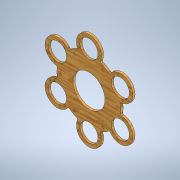
# Autodesk Inventor part: AmmoHolder
Saved by Autodesk Inventor 2020.2 (Build 242310000, 310)
## iProperties
Created: 2019-11-06
Part Number: AmmoHolder
Material: Plywood, Finish
Document SubType Name: Modeling
Designer: Paul Lefeuvre
Density: 0.552 g/cm^3
Appearance: Plywood - New
Mass: 279.601 g
Surface Area: 1409.01 cm^2
Volume: 506.524 cm^3
Author: Paul Lefeuvre
Autodesk Inventor part; units mm, degrees
ref_plane "YZ Plane" through (0, 0, 0) normal (1, 0, 0) x (0, 1, 0)
ref_plane "XZ Plane" through (0, 0, 0) normal (0, 1, 0) x (-1, 0, 0)
ref_plane "XY Plane" through (0, 0, 0) normal (0, 0, 1) x (1, 0, 0)
sketch "Sketch3" plane through (0, 0, 0) normal (0, 0, 1) x (1, 0, 0)
  circle A0 centre (0, 0) radius 191.2 construction
  circle A1 centre (0, 153.1) radius 37.5 construction
  circle A2 centre (0, 153.1) radius 38.1
  line L0 (0, 0) -> (0, 212.7207) construction
  arc A3 (48.5367, 131.5641) -> (-48.5367, 131.5641) centre (0, 153.1) ccw
  arc A4 (-51.2104, 124.91) -> (-48.5367, 131.5641) centre (-53.1071, 129.5363) ccw
  arc A5 (48.5367, 131.5641) -> (51.2104, 124.91) centre (53.1071, 129.5363) ccw
  circle A6 centre (-132.5885, 76.55) radius 38.1
  arc A7 (-89.6695, 107.8161) -> (-138.2062, 23.748) centre (-132.5885, 76.55) ccw
  arc A8 (-133.7804, 18.1055) -> (-138.2062, 23.748) centre (-138.7352, 18.7761) ccw
  arc A9 (-89.6695, 107.8161) -> (-82.57, 106.8045) centre (-85.6282, 110.7602) ccw
  circle A10 centre (-132.5885, -76.55) radius 38.1
  arc A11 (-138.2062, -23.748) -> (-89.6695, -107.8161) centre (-132.5885, -76.55) ccw
  arc A12 (-82.57, -106.8045) -> (-89.6695, -107.8161) centre (-85.6282, -110.7602) ccw
  arc A13 (-138.2062, -23.748) -> (-133.7804, -18.1055) centre (-138.7352, -18.7761) ccw
  circle A14 centre (0, -153.1) radius 38.1
  arc A15 (-48.5367, -131.5641) -> (48.5367, -131.5641) centre (0, -153.1) ccw
  arc A16 (51.2104, -124.91) -> (48.5367, -131.5641) centre (53.1071, -129.5363) ccw
  arc A17 (-48.5367, -131.5641) -> (-51.2104, -124.91) centre (-53.1071, -129.5363) ccw
  circle A18 centre (132.5885, -76.55) radius 38.1
  arc A19 (89.6695, -107.8161) -> (138.2062, -23.748) centre (132.5885, -76.55) ccw
  arc A20 (133.7804, -18.1055) -> (138.2062, -23.748) centre (138.7352, -18.7761) ccw
  arc A21 (89.6695, -107.8161) -> (82.57, -106.8045) centre (85.6282, -110.7602) ccw
  circle A22 centre (132.5885, 76.55) radius 38.1
  arc A23 (138.2062, 23.748) -> (89.6695, 107.8161) centre (132.5885, 76.55) ccw
  arc A24 (82.57, 106.8045) -> (89.6695, 107.8161) centre (85.6282, 110.7602) ccw
  arc A25 (138.2062, 23.748) -> (133.7804, 18.1055) centre (138.7352, 18.7761) ccw
  arc A26 (-51.2104, 124.91) -> (-82.57, 106.8045) centre (0, 0) ccw
  arc A27 (82.57, 106.8045) -> (51.2104, 124.91) centre (0, 0) ccw
  arc A28 (133.7804, -18.1055) -> (133.7804, 18.1055) centre (0, 0) ccw
  arc A29 (51.2104, -124.91) -> (82.57, -106.8045) centre (0, 0) ccw
  arc A30 (-82.57, -106.8045) -> (-51.2104, -124.91) centre (0, 0) ccw
  arc A31 (-133.7804, 18.1055) -> (-133.7804, -18.1055) centre (0, 0) ccw
  circle A32 centre (41.5415, 141.1) radius 3.3
  line L1 (0, 153.1) -> (41.5415, 141.1) construction
  circle A33 centre (41.5415, 165.1) radius 3.3
  line L2 (0, 153.1) -> (41.5415, 165.1) construction
  line L3 (41.5415, 141.1) -> (41.5415, 165.1) construction
  circle A34 centre (-41.5415, 141.1) radius 3.3
  circle A35 centre (-41.5415, 165.1) radius 3.3
  circle A36 centre (-163.7516, 46.574) radius 3.3
  circle A37 centre (-142.9669, 34.574) radius 3.3
  circle A38 centre (-122.21, 118.526) radius 3.3
  circle A39 centre (-101.4254, 106.526) radius 3.3
  circle A40 centre (-122.21, -118.526) radius 3.3
  circle A41 centre (-101.4254, -106.526) radius 3.3
  circle A42 centre (-163.7516, -46.574) radius 3.3
  circle A43 centre (-142.9669, -34.574) radius 3.3
  circle A44 centre (41.5415, -165.1) radius 3.3
  circle A45 centre (41.5415, -141.1) radius 3.3
  circle A46 centre (-41.5415, -165.1) radius 3.3
  circle A47 centre (-41.5415, -141.1) radius 3.3
  circle A48 centre (163.7516, -46.574) radius 3.3
  circle A49 centre (142.9669, -34.574) radius 3.3
  circle A50 centre (122.21, -118.526) radius 3.3
  circle A51 centre (101.4254, -106.526) radius 3.3
  circle A52 centre (122.21, 118.526) radius 3.3
  circle A53 centre (101.4254, 106.526) radius 3.3
  circle A54 centre (163.7516, 46.574) radius 3.3
  circle A55 centre (142.9669, 34.574) radius 3.3
  circle A56 centre (0, 0) radius 100 construction
  circle A57 centre (0, 0) radius 72.5 construction
  circle A58 centre (0, 0) radius 67.5
  line L4 (0, 0) -> (-241.025, 0) construction
  circle A59 centre (-120, 0) radius 3.9
  line L5 (0, 0) -> (-120.5125, -208.7337) construction
  circle A60 centre (-60, -103.923) radius 3.9
  line L6 (0, 0) -> (120.5125, -208.7337) construction
  circle A61 centre (60, -103.923) radius 3.9
  line L7 (0, 0) -> (241.025, 0) construction
  circle A62 centre (120, 0) radius 3.9
  line L8 (0, 0) -> (120.5125, 208.7337) construction
  circle A63 centre (60, 103.923) radius 3.9
  line L9 (0, 0) -> (-120.5125, 208.7337) construction
  circle A64 centre (-60, 103.923) radius 3.9
  point P0 (-34.2525, 136.4155)
  point P1 (34.2525, 136.4155)
  point P2 (-135.2655, 38.5442)
  point P3 (-101.013, 97.8713)
  point P4 (-101.013, -97.8713)
  point P5 (-135.2655, -38.5442)
  point P6 (34.2525, -136.4155)
  point P7 (-34.2525, -136.4155)
  point P8 (135.2655, -38.5442)
  point P9 (101.013, -97.8713)
  point P10 (101.013, 97.8713)
  point P11 (135.2655, 38.5442)
  dimension "d0" = 382.4
  dimension "d1" = 75
  dimension "d2" = 0.6
  dimension "d4" = 15
  dimension "d5" = 5
  dimension "d11" = 360
  dimension "d23" = 135
  dimension "d24" = 6.6
  dimension "d26" = 43.24
  dimension "d27" = 6.6
  dimension "d28" = 43.24
  dimension "d29" = 24
  dimension "d32" = 360
  dimension "d34" = 200
  dimension "d35" = 145
  dimension "d36" = 5
  dimension "d37" = 7.8
  dimension "d38" = 120
  dimension "d41" = 360
  constraints: 65 centre point, 60 point on circle, 20 end point, 7 point on line, 5 tangent, 4 coincident, 2 symmetric about line, 2 vertical, 1 equal radius, 1 horizontal, 161 other
  measures "d0" diameter of A0
  measures "d1" diameter of A1
  measures "d2" radial gap between concentric circles of A1 A2
  measures "d4" radial gap between concentric circles of A2 A3
  measures "d5" radius of A4
  measures "d23" radius of A27
  measures "d24" diameter of A32
  measures "d26" distance of L1.start L1.end
  measures "d27" diameter of A33
  measures "d28" distance of L1.start L2.end
  measures "d29" distance of L1.end L2.end
  measures "d34" diameter of A56
  measures "d35" diameter of A57
  measures "d36" radial gap between concentric circles of A57 A58
  measures "d37" diameter of A59
  measures "d38" distance of point (0, 0) A59.centre
extrude "Extrusion1" add sketch "Sketch3" along normal blind 9
body "Solid1"
